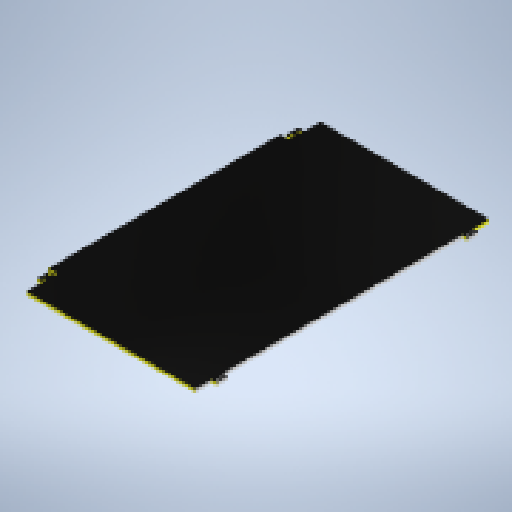
# Autodesk Inventor part: pantalla
Saved by Autodesk Inventor 2023 (Build 270158000, 158)
## iProperties
Created: 2023-05-12
Part Number: pantalla
Material: Genérico
Document SubType Name: Modeling
Designer: sergi
Density: 1 g/cm^3
Appearance: Valor por defecto
Author: sergi
Autodesk Inventor part; units mm, degrees
ref_plane "YZ Plane" through (0, 0, 0) normal (1, 0, 0) x (0, 1, 0)
ref_plane "XZ Plane" through (0, 0, 0) normal (0, 1, 0) x (-1, 0, 0)
ref_plane "XY Plane" through (0, 0, 0) normal (0, 0, 1) x (1, 0, 0)
sketch "Boceto3" plane through (0, 0, 0) normal (0, 1, 0) x (-1, 0, 0)
  line L0 (-109, -180) -> (109, -180)
  line L1 (109, -180) -> (109, 180)
  line L2 (109, 180) -> (-109, 180)
  line L3 (-109, 180) -> (-109, -180)
  line L4 (-109, -180) -> (109, 180) construction
  line L5 (109, -180) -> (-109, 180) construction
  line L6 (0, 180) -> (103.5, 180)
  line L7 (109, 180) -> (97.75, 180)
  line L8 (97.75, 180) -> (97.75, 160)
  line L9 (97.75, 180) -> (117.75, 180) construction
  line L10 (97.75, 160) -> (105.25, 160)
  line L11 (105.25, 160) -> (105.25, 145)
  line L12 (105.25, 145) -> (97.75, 145)
  line L13 (97.75, 145) -> (97.75, 142)
  line L14 (97.75, 142) -> (109, 142)
  line L15 (109, -180) -> (97.75, -180)
  line L16 (97.75, -180) -> (97.75, -160)
  line L17 (97.75, -180) -> (117.75, -180) construction
  line L18 (97.75, -160) -> (105.25, -160)
  line L19 (105.25, -160) -> (105.25, -145)
  line L20 (105.25, -145) -> (97.75, -145)
  line L21 (97.75, -145) -> (97.75, -142)
  line L22 (97.75, -142) -> (109, -142)
  line L23 (-109, 180) -> (-102.7, 180)
  line L24 (-109, 180) -> (-109, 160)
  line L25 (-109, 160) -> (-115.3, 160)
  line L26 (-109, 160) -> (-109, 146.9)
  line L27 (-115.3, 146.9) -> (-109, 146.9)
  line L28 (-109, 146.9) -> (-109, -180)
  line L29 (-102.7, -180) -> (-102.7, -160)
  line L30 (-102.7, -180) -> (-82.7, -180) construction
  line L31 (-109, -160) -> (-115.3, -160)
  line L32 (-109, -160) -> (-109, -146.9)
  line L33 (-115.3, -146.9) -> (-109, -146.9)
  line L34 (-115.3, 160) -> (-115.3, 146.9)
  line L35 (-115.3, -146.9) -> (-115.3, -160)
  point P0 (0, 0)
  point P1 (-109, -180)
  dimension "d27" = 218
  dimension "d28" = 360
  dimension "d33" = 11.25
  dimension "d34" = 20
  dimension "d35" = 90
  dimension "d36" = 7.5
  dimension "d37" = 15
  dimension "d38" = 7.5
  dimension "d39" = 3
  dimension "d40" = 11.25
  dimension "d41" = 20
  dimension "d42" = 90
  dimension "d43" = 15
  dimension "d44" = 3
  dimension "d45" = 6.3
  dimension "d46" = 20
  dimension "d47" = 90
  dimension "d48" = 13.1
  dimension "d49" = 90
  dimension "d50" = 20
  dimension "d51" = 90
  dimension "d52" = 13.1
  constraints: 72 end point, 14 perpendicular, 12 point on line, 4 horizontal, 4 parallel, 3 midpoint, 3 vertical, 1 collinear
  measures "d27" distance of L2.end L1.end
  measures "d28" distance of L1.end L0.end
  measures "d33" distance of L1.end L7.end
  measures "d34" distance of L7.end L8.end
  measures "d35" angle of L8 L9
  measures "d36" distance of L8.end L10.end
  measures "d37" distance of L10.end L11.end
  measures "d38" distance of L11.end L12.end
  measures "d39" distance of L12.end L13.end
  measures "d40" distance of L0.end L15.end
  measures "d41" distance of L15.end L16.end
  measures "d42" angle of L17 L16
  measures "d43" distance of L18.end L19.end
  measures "d44" distance of L20.end L21.end
  measures "d45" distance of L23.end L2.end
  measures "d46" distance of L24.start L24.end
  measures "d47" angle of L23 L24
  measures "d48" distance of L26.start L26.end
  measures "d49" angle of L27 L26
  measures "d50" distance of L29.start L29.end
  measures "d51" angle of L30 L29
  measures "d52" distance of L32.start L32.end
extrude "Extrusión2" add sketch "Boceto3" along normal blind 3.6 contours L3 L2 L8 L10 L11 L12 L13 L14 L1 L22 L21 L20 L19 L18 L16 L0 | L31 L35 L33 L3 | L27 L34 L25 L3
sketch "Boceto4" plane through (0, 3.6, 0) normal (0, 1, 0) x (1, 0, 0)
  line L0 (-105.25, -145) -> (-105.25, -160) projected
  line L1 (-105.25, -160) -> (-97.75, -160) projected
  line L2 (-97.75, -145) -> (-105.25, -145) projected
  point P0 (0, 0)
  point P1 (-100.65, -156.7)
  point P2 (-100.65, -148.3)
  dimension "d55" = 4.6
  dimension "d56" = 3.3
  dimension "d73" = 3.3
  dimension "d74" = 4.6
  measures "d55" distance from line of L0 point (-100.65, -156.7)
  measures "d56" distance from line of L1 point (-100.65, -156.7)
  measures "d73" distance from line of L2 point (-100.65, -148.3)
  measures "d74" distance from line of L0 point (-100.65, -148.3)
hole "Agujero1" at (-100.65, 3.6, 156.7) at (-100.65, 3.6, 148.3) direction (0, -1, 0) diameter 3.3 end through all
mirror "Simetría1" about plane through (0, 0, 0) normal (0, 0, 1) of "Agujero1"
sketch "Boceto6" plane through (0, 3.6, 0) normal (0, 1, 0) x (1, 0, 0)
  line L0 (109, -160) -> (115.3, -160) projected
  line L1 (109, 160) -> (109, 180) projected
  line L2 (115.3, -146.9) -> (109, -146.9) projected
  line L3 (115.3, -156.3) -> (111.9, -156.3)
  line L4 (111.9, -156.3) -> (111.9, -150.6)
  circle A0 centre (111.9, -156.3) radius 1.2
  circle A1 centre (111.9, -150.6) radius 1.2
  point P0 (0, 0)
  point P1 (105.6, -156.3)
  point P2 (102.7, -160)
  point P3 (105.6, -150.6)
  point P4 (102.7, -146.9)
  dimension "d75" = 3.7
  dimension "d76" = 3.4
  dimension "d77" = 3.7
  dimension "d78" = 3.4
  dimension "d95" = 3.4
  dimension "d96" = 2.4
  dimension "d97" = 2.4
  constraints: 4 end point, 2 centre point, 2 coincident, 1 horizontal, 1 perpendicular, 1 other
  measures "d75" distance from line of L0 point (105.6, -156.3)
  measures "d77" distance from line of L2 point (105.6, -150.6)
  measures "d95" distance of L3.start L3.end
  measures "d96" diameter of A0
  measures "d97" diameter of A1
hole "Agujero3" at (111.9, 3.6, 156.3) at (111.9, 3.6, 150.6) direction (0, -1, 0) diameter 2.4 end through all
mirror "Simetría2" about plane through (0, 0, 0) normal (0, 0, 1) of "Agujero3"
equation "\"d57\" = d73"
